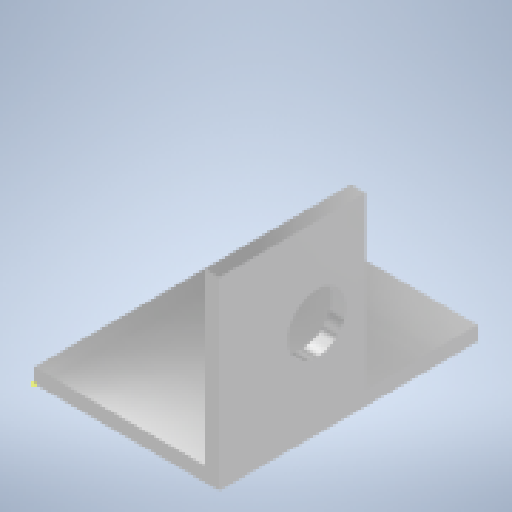
# Autodesk Inventor part: P005
Saved by Autodesk Inventor 2023 (Build 270158000, 158)
## iProperties
Created: 2022-09-15
Part Number: P005
Material: Aluminum 6061
Document SubType Name: Modeling
Designer: D.C. Eksteen
Density: 2.7 g/cm^3
Appearance: Aluminum - Flat
Author: D.C. Eksteen
Title: MOTOR MOUNT
Autodesk Inventor part; units mm, degrees
ref_plane "YZ Plane" through (0, 0, 0) normal (1, 0, 0) x (0, 1, 0)
ref_plane "XZ Plane" through (0, 0, 0) normal (0, 1, 0) x (-1, 0, 0)
ref_plane "XY Plane" through (0, 0, 0) normal (0, 0, 1) x (1, 0, 0)
sketch "Sketch1" plane through (0, 0, 0) normal (0, 0, 1) x (1, 0, 0)
  point P0 (0, 0)
sketch "Sketch2" plane through (0, 0, 0) normal (0, 0, 1) x (1, 0, 0)
  line L0 (0, 0) -> (76, 0)
  line L1 (76, 0) -> (76, 76)
  line L2 (76, 76) -> (0, 76)
  line L3 (0, 76) -> (0, 0)
  line L4 (70, 6) -> (6, 6)
  line L5 (6, 6) -> (6, 70)
  line L6 (6, 70) -> (70, 70)
  line L7 (70, 70) -> (70, 6)
  line L8 (6, 6) -> (0, 6)
  line L9 (70, 70) -> (70, 76)
  dimension "d0" = 76
  dimension "d1" = 76
  dimension "d2" = 6
  constraints: 20 end point, 4 parallel, 4 perpendicular, 2 point on line, 1 horizontal, 3 other
  measures "d0" distance of L2.end L1.end
  measures "d1" distance of L1.end L0.end
  measures "d2" distance between parallel lines of L0 L4
extrude "Extrusion1" add sketch "Sketch2" against normal blind 106 contours L3 L8 L4 L7 L9 L2 L1 L0
sketch "Sketch3" plane through (76, 76, 0) normal (1, 0, 0) x (0, 0, -1)
  line L0 (106, 0) -> (106, -76) projected
  line L1 (0, 0) -> (106, 0) projected
  line L2 (0, -76) -> (0, 0) projected
  circle A0 centre (40, -36.5) radius 12
  line L3 (0, -76) -> (106, -76) projected
  dimension "d6" = 24
  dimension "d7" = 40
  constraints: 1 centre point
  measures "d6" diameter of A0
  measures "d7" distance from line of L2 A0.centre
extrude "Extrusion2" cut sketch "Sketch3" against normal blind 76 contours A0
sketch "Sketch5" plane through (70, 76, -106) normal (-1, 0, 0) x (0, 0, 1)
  line L0 (0, -70) -> (106, -70) projected
  line L1 (106, 0) -> (0, 0) projected
  line L2 (106, -70) -> (46, -70)
  line L3 (46, -70) -> (46, 0)
  line L4 (46, 0) -> (106, 0)
  line L5 (106, 0) -> (106, -70)
  line L6 (0, -70) -> (0, 0) projected
  line L7 (0, 0) -> (46, 0)
  line L8 (46, 0) -> (46, -70)
  line L9 (46, -70) -> (0, -70)
  line L10 (0, -70) -> (0, 0)
  point P0 (106, -76)
  dimension "d23" = 60
  constraints: 16 end point, 4 parallel, 2 horizontal, 2 perpendicular, 1 point on line
  measures "d23" distance of L3.end L4.end
extrude "Extrusion3" cut sketch "Sketch5" against normal blind 10 contours L6 L1 L3 L0
body "Solid1"
